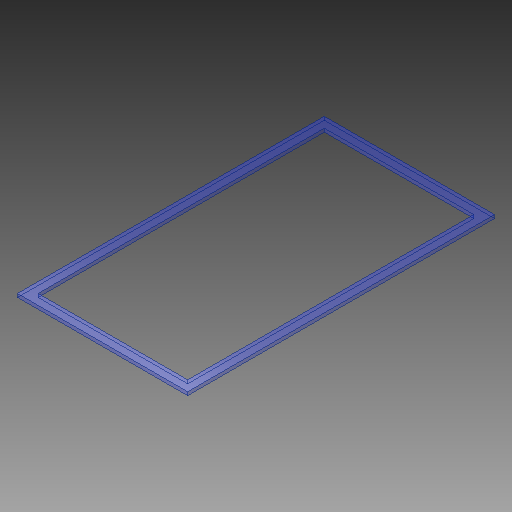
# Autodesk Inventor part: sb_bottom
Saved by Autodesk Inventor 2018.1 (Build 221171000, 171)
## iProperties
Created: 2017-08-17
Part Number: sb_bottom
Material: PVC-Piping
Document SubType Name: Modeling
Designer: Tom
Density: 1.4 g/cm^3
Appearance: Clear - Blue
Author: Tom
Autodesk Inventor part; units mm, degrees
ref_plane "YZ Plane" through (0, 0, 0) normal (1, 0, 0) x (0, 1, 0)
ref_plane "XZ Plane" through (0, 0, 0) normal (0, 1, 0) x (-1, 0, 0)
ref_plane "XY Plane" through (0, 0, 0) normal (0, 0, 1) x (1, 0, 0)
sketch "Sketch1" plane through (0, 0, 0) normal (0, 1, 0) x (-1, 0, 0)
  line L0 (130, 230) -> (-130, 230)
  line L1 (-130, 230) -> (-130, -230)
  line L2 (-130, -230) -> (130, -230)
  line L3 (130, -230) -> (130, 230)
  line L4 (130, 230) -> (-130, -230) construction
  line L5 (-130, 230) -> (130, -230) construction
  line L6 (124.5, -224.5) -> (-124.5, -224.5)
  line L7 (-124.5, -224.5) -> (-124.5, 224.5)
  line L8 (-124.5, 224.5) -> (124.5, 224.5)
  line L9 (124.5, 224.5) -> (124.5, -224.5)
  line L10 (124.5, -224.5) -> (-124.5, 224.5) construction
  line L11 (-124.5, -224.5) -> (124.5, 224.5) construction
  line L12 (-109.5, 209.5) -> (109.5, 209.5)
  line L13 (109.5, 209.5) -> (109.5, -209.5)
  line L14 (109.5, -209.5) -> (-109.5, -209.5)
  line L15 (-109.5, -209.5) -> (-109.5, 209.5)
  line L16 (-109.5, 209.5) -> (109.5, -209.5) construction
  line L17 (109.5, 209.5) -> (-109.5, -209.5) construction
  point P0 (0, 0)
  dimension "d0" = 260
  dimension "d1" = 460
  dimension "d8" = 249
  dimension "d9" = 449
  dimension "d10" = 219
  dimension "d11" = 419
  constraints: 36 end point, 6 midpoint, 6 parallel, 3 horizontal, 3 perpendicular
  measures "d0" distance of L2.end L1.end
  measures "d1" distance of L1.end L0.end
  measures "d8" distance of L7.end L8.end
  measures "d9" distance of L6.end L7.end
  measures "d10" distance of L13.end L14.end
  measures "d11" distance of L12.end L13.end
extrude "Extrusion3" add sketch "Sketch1" along normal blind 5 contours L6 L7 L8 L9
equation "\"d0\" = boxl + 2 * pvct"
equation "\"d1\" = boxw + 2 * pvct"
equation "\"d8\" = boxl - 2 * play"
equation "\"d9\" = boxw - 2 * play"
equation "\"d10\" = boxl - 2 * play - 2 * supporth"
equation "\"d11\" = boxw - 2 * play - 2 * supporth"
equation "\"d12\" = pvct"
equation "\"solhole\" = 3"
equation "\"solholespacing\" = 16"
equation "\"ssolw\" = 63"
equation "\"bsoll\" = 126"
equation "\"bsolw\" = 91"
equation "\"bsolh\" = 126"
equation "\"tapl\" = 31"
equation "\"tl\" = 32"
equation "\"eloboww\" = 25"
equation "\"pvct\" = 5"
equation "\"boxh\" = 258"
equation "\"supporth\" = 15"
equation "\"play\" = 0.5"
equation "\"arw\" = 54"
equation "\"arl\" = 102"
equation "\"psuh\" = 85"
equation "\"screenw\" = 197"
equation "\"screenl\" = 115"
equation "\"pcbw\" = 76"
equation "\"pcbl\" = 86"
equation "\"pcbh\" = 46"
equation "\"seph\" = 105"
equation "\"diaetape\" = 25"
equation "\"diaload\" = 16"
equation "\"diapower\" = 16"
equation "\"diaph\" = 32"
equation "\"distbubblewater\" = 82"
equation "\"distpumps\" = 75"
equation "\"waterouter\" = 39"
equation "\"waterinner\" = 28"
equation "\"pumpinner\" = 16"
equation "\"pumpouter\" = 25"
equation "\"airoutinner\" = 28"
equation "\"airoutouter\" = 39"
equation "\"airinouter\" = 39"
equation "\"airininner\" = 28"
equation "\"diapowerouter\" = 25"
equation "\"dialoadouter\" = 25"
equation "\"diaetapeouter\" = 36"
equation "\"diaphouter\" = 48"
equation "\"boxl\" = 250"
equation "\"boxw\" = 450"
body "Solid2"
